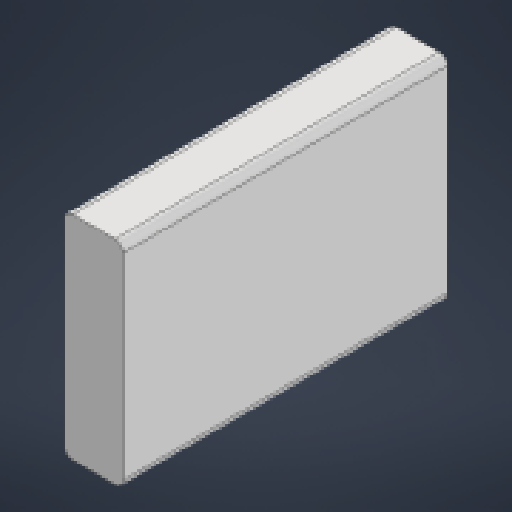
# Autodesk Inventor part: USRPB210
Saved by Autodesk Inventor 2023.4 (Build 274418000, 418)
## iProperties
Created: 2025-10-22
Part Number: USRPB210
Material: Generic
Document SubType Name: Modeling
Designer: Malthe Sennels
Density: 1 g/cm^3
Appearance: Default
Author: Malthe Sennels
Autodesk Inventor part; units mm, degrees
ref_plane "YZ Plane" through (0, 0, 0) normal (1, 0, 0) x (0, 1, 0)
ref_plane "XZ Plane" through (0, 0, 0) normal (0, 1, 0) x (-1, 0, 0)
ref_plane "XY Plane" through (0, 0, 0) normal (0, 0, 1) x (1, 0, 0)
sketch "Sketch1" plane through (0, 0, 0) normal (0, 0, 1) x (1, 0, 0)
  line L0 (-10.5, 52.5) -> (10.5, 52.5)
  line L1 (14.5, 48.5) -> (14.5, -48.5)
  line L2 (10.5, -52.5) -> (-10.5, -52.5)
  line L3 (-14.5, -48.5) -> (-14.5, 48.5)
  line L4 (-14.5, 52.5) -> (14.5, -52.5) construction
  line L5 (14.5, 52.5) -> (-14.5, -52.5) construction
  arc A0 (14.5, 48.5) -> (10.5, 52.5) centre (10.5, 48.5) ccw
  arc A1 (-10.5, 52.5) -> (-14.5, 48.5) centre (-10.5, 48.5) ccw
  arc A2 (-14.5, -48.5) -> (-10.5, -52.5) centre (-10.5, -48.5) ccw
  arc A3 (10.5, -52.5) -> (14.5, -48.5) centre (10.5, -48.5) ccw
  point P0 (0, 0)
  dimension "d0" = 29
  dimension "d1" = 105
  dimension "d2" = 4
  constraints: 12 end point, 8 point on circle, 8 point on line, 8 tangent, 4 centre point, 3 equal radius, 2 midpoint, 2 parallel, 1 horizontal, 1 perpendicular
  measures "d0" distance of L4.end L5.end
  measures "d1" distance of L5.start L4.end
  measures "d2" radius of A0
extrude "Extrusion1" add sketch "Sketch1" along normal blind 160
body "Solid1"
